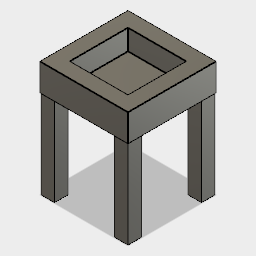
box_model_v1 (Autodesk Fusion 360 design; units mm, degrees)
Autodesk Fusion 360 part; units mm, degrees
sketch "Sketch1" plane through (0, 0, 0) normal (0, 1, 0) x (1, 0, 0)
  line L0 (14.6204, -9.8795) -> (79.6204, -9.8795)
  line L1 (79.6204, -9.8795) -> (79.6204, -74.8795)
  line L2 (79.6204, -74.8795) -> (14.6204, -74.8795)
  line L3 (14.6204, -74.8795) -> (14.6204, -9.8795)
  line L4 (68.3204, -63.5795) -> (25.9204, -63.5795)
  line L5 (25.9204, -63.5795) -> (25.9204, -21.1795)
  line L6 (25.9204, -21.1795) -> (68.3204, -21.1795)
  line L7 (68.3204, -21.1795) -> (68.3204, -63.5795)
  line L8 (15.1804, -10.4395) -> (25.1804, -10.4395)
  line L9 (25.1804, -10.4395) -> (25.1804, -20.4395)
  line L10 (25.1804, -20.4395) -> (15.1804, -20.4395)
  line L11 (15.1804, -20.4395) -> (15.1804, -10.4395)
  line L12 (79.0604, -10.4395) -> (69.0604, -10.4395)
  line L13 (69.0604, -10.4395) -> (69.0604, -20.4395)
  line L14 (69.0604, -20.4395) -> (79.0604, -20.4395)
  line L15 (79.0604, -20.4395) -> (79.0604, -10.4395)
  line L16 (15.1804, -74.3195) -> (25.1804, -74.3195)
  line L17 (25.1804, -74.3195) -> (25.1804, -64.3195)
  line L18 (25.1804, -64.3195) -> (15.1804, -64.3195)
  line L19 (15.1804, -64.3195) -> (15.1804, -74.3195)
  line L20 (79.0604, -74.3195) -> (69.0604, -74.3195)
  line L21 (69.0604, -74.3195) -> (69.0604, -64.3195)
  line L22 (69.0604, -64.3195) -> (79.0604, -64.3195)
  line L23 (79.0604, -64.3195) -> (79.0604, -74.3195)
  line L24 (17.6804, -12.9395) -> (22.6804, -12.9395)
  line L25 (22.6804, -12.9395) -> (22.6804, -17.9395)
  line L26 (22.6804, -17.9395) -> (17.6804, -17.9395)
  line L27 (17.6804, -17.9395) -> (17.6804, -12.9395)
  line L28 (76.5604, -12.9395) -> (71.5604, -12.9395)
  line L29 (71.5604, -12.9395) -> (71.5604, -17.9395)
  line L30 (71.5604, -17.9395) -> (76.5604, -17.9395)
  line L31 (76.5604, -17.9395) -> (76.5604, -12.9395)
  line L32 (17.6804, -66.8195) -> (17.6804, -71.8195)
  line L33 (17.6804, -71.8195) -> (22.6804, -71.8195)
  line L34 (22.6804, -71.8195) -> (22.6804, -66.8195)
  line L35 (22.6804, -66.8195) -> (17.6804, -66.8195)
  line L36 (76.5604, -66.8195) -> (76.5604, -71.8195)
  line L37 (76.5604, -71.8195) -> (71.5604, -71.8195)
  line L38 (71.5604, -71.8195) -> (71.5604, -66.8195)
  line L39 (71.5604, -66.8195) -> (76.5604, -66.8195)
  dimension "d1" = 65
  dimension "d2" = 65
  dimension "d6" = 11.3
  dimension "d8" = 10
  dimension "d9" = 10
  dimension "d10" = 10
  dimension "d11" = 10
  dimension "d12" = 10
  dimension "d13" = 10
  dimension "d14" = 10
  dimension "d15" = 10
  dimension "d16" = 2.5
  dimension "d17" = 2.5
  dimension "d18" = 2.5
  dimension "d19" = 2.5
  measures "d1" distance of L0.start L0.end
  measures "d2" distance of L0.start L2.end
  measures "d8" distance of L8.start L8.end
  measures "d9" distance of L8.start L10.end
  measures "d10" distance of L12.start L12.end
  measures "d11" distance of L12.start L14.end
  measures "d12" distance of L16.start L16.end
  measures "d13" distance of L16.start L18.end
  measures "d14" distance of L20.start L20.end
  measures "d15" distance of L20.start L22.end
extrude "Extrude1" add sketch "Sketch1" along normal blind 5 contours L4 L5 L6 L7 makes body 1
extrude "Extrude2" add sketch "Sketch1" along normal blind 20 contours L0 L1 L2 L3 | L8 L9 L10 L11 | L12 L13 L14 L15 | L16 L17 L18 L19 | L20 L21 L22 L23 | L24 L25 L26 L27 | L28 L29 L30 L31 | L32 L33 L34 L35 | L36 L37 L38 L39 bodies 1
extrude "Extrude3" cut sketch "Sketch1" along normal blind 3 contours L24 L25 L26 L27 | L28 L29 L30 L31 | L32 L33 L34 L35 | L36 L37 L38 L39 bodies 1
extrude "Extrude4" cut sketch "Sketch1" along normal blind 1 contours L8 L9 L10 L11 | L12 L13 L14 L15 | L16 L17 L18 L19 | L20 L21 L22 L23 bodies 1
fillet "Fillet1" radius 0.3 20 edges at (47.1204, 20, 74.8795) (79.6204, 10, 74.8795) (79.6204, 20, 42.3795) (79.6204, 10, 9.8795) (47.1204, 20, 9.8795) (14.6204, 20, 42.3795) (47.1204, 20, 63.5795) (25.9204, 20, 42.3795) (47.1204, 20, 21.1795) (68.3204, 20, 42.3795) (47.1204, 5, 63.5795) (25.9204, 5, 42.3795) (47.1204, 5, 21.1795) (68.3204, 12.5, 21.1795) (68.3204, 5, 42.3795) (68.3204, 12.5, 63.5795) (25.9204, 12.5, 63.5795) (25.9204, 12.5, 21.1795) (14.6204, 10, 74.8795) (14.6204, 10, 9.8795) on bodies 1
copy_body "Body->Comp1" bodies 1 removing the originals makes body 2 in component "Motor Housing"
sketch "Sketch2" plane through (0, 0, 0) normal (0, 1, 0) x (1, 0, 0) in component "Motor Housing"
  line L0 (100.3048, -10.6918) -> (166.3048, -10.6918)
  line L1 (166.3048, -10.6918) -> (166.3048, -20.6918)
  line L2 (166.3048, -20.6918) -> (100.3048, -20.6918)
  line L3 (100.3048, -20.6918) -> (100.3048, -10.6918)
  line L4 (100.3048, -30.5722) -> (166.3048, -30.5722)
  line L5 (166.3048, -30.5722) -> (166.3048, -40.5722)
  line L6 (166.3048, -40.5722) -> (100.3048, -40.5722)
  line L7 (100.3048, -40.5722) -> (100.3048, -30.5722)
  line L8 (100.3048, -49.9678) -> (166.3048, -49.9678)
  line L9 (166.3048, -49.9678) -> (166.3048, -59.9678)
  line L10 (166.3048, -59.9678) -> (100.3048, -59.9678)
  line L11 (100.3048, -59.9678) -> (100.3048, -49.9678)
  line L12 (100.3048, -70.0907) -> (166.3048, -70.0907)
  line L13 (166.3048, -70.0907) -> (166.3048, -80.0907)
  line L14 (166.3048, -80.0907) -> (100.3048, -80.0907)
  line L15 (100.3048, -80.0907) -> (100.3048, -70.0907)
  dimension "d32" = 66
  dimension "d33" = 10
  dimension "d34" = 10
  dimension "d35" = 10
  dimension "d36" = 10
  measures "d32" distance of L0.start L0.end
  measures "d33" distance of L0.start L2.end
  measures "d34" distance of L4.start L6.end
  measures "d35" distance of L8.start L10.end
  measures "d36" distance of L12.start L14.end
extrude "Extrude1'" add sketch "Sketch2" along normal blind 10 separate body makes body 3 at (122.3048, 3.3333, 49.9678) makes body 4 at (122.3048, 3.3333, 30.5722) makes body 5 at (122.3048, 3.3333, 70.0907) makes body 6 at (122.3048, 3.3333, 10.6918) in component "Motor Housing"
sketch "Sketch3" plane through (166.3048, 0, 0) normal (1, 0, 0) x (0, 0, -1) in component "Motor Housing"
  line L0 (-80.0907, 0) -> (-70.0907, 0)
  line L1 (-70.0907, 0) -> (-70.0907, 10)
  line L2 (-70.0907, 10) -> (-80.0907, 10)
  line L3 (-80.0907, 10) -> (-80.0907, 0)
  line L4 (-77.5907, 2.5) -> (-72.5907, 2.5)
  line L5 (-72.5907, 2.5) -> (-72.5907, 7.5)
  line L6 (-72.5907, 7.5) -> (-77.5907, 7.5)
  line L7 (-77.5907, 7.5) -> (-77.5907, 2.5)
  dimension "d39" = 2.5
sketch "Sketch4" plane through (166.3048, 0, 0) normal (1, 0, 0) x (0, 0, -1) in component "Motor Housing"
  line L0 (-59.9678, 0) -> (-49.9678, 0)
  line L1 (-49.9678, 0) -> (-49.9678, 10)
  line L2 (-49.9678, 10) -> (-59.9678, 10)
  line L3 (-59.9678, 10) -> (-59.9678, 0)
  line L4 (-57.4678, 2.5) -> (-52.4678, 2.5)
  line L5 (-52.4678, 2.5) -> (-52.4678, 7.5)
  line L6 (-52.4678, 7.5) -> (-57.4678, 7.5)
  line L7 (-57.4678, 7.5) -> (-57.4678, 2.5)
  dimension "d40" = 2.5
sketch "Sketch5" plane through (166.3048, 0, 0) normal (1, 0, 0) x (0, 0, -1) in component "Motor Housing"
  line L0 (-40.5722, 0) -> (-30.5722, 0)
  line L1 (-30.5722, 0) -> (-30.5722, 10)
  line L2 (-30.5722, 10) -> (-40.5722, 10)
  line L3 (-40.5722, 10) -> (-40.5722, 0)
  line L4 (-38.0722, 2.5) -> (-33.0722, 2.5)
  line L5 (-33.0722, 2.5) -> (-33.0722, 7.5)
  line L6 (-33.0722, 7.5) -> (-38.0722, 7.5)
  line L7 (-38.0722, 7.5) -> (-38.0722, 2.5)
  dimension "d41" = 2.5
sketch "Sketch6" plane through (166.3048, 0, 0) normal (1, 0, 0) x (0, 0, -1) in component "Motor Housing"
  line L0 (-20.6918, 0) -> (-10.6918, 0)
  line L1 (-10.6918, 0) -> (-10.6918, 10)
  line L2 (-10.6918, 10) -> (-20.6918, 10)
  line L3 (-20.6918, 10) -> (-20.6918, 0)
  line L4 (-18.1918, 2.5) -> (-13.1918, 2.5)
  line L5 (-13.1918, 2.5) -> (-13.1918, 7.5)
  line L6 (-13.1918, 7.5) -> (-18.1918, 7.5)
  line L7 (-18.1918, 7.5) -> (-18.1918, 2.5)
  dimension "d42" = 2.5
extrude "Extrude2'" add sketch "Sketch5" sketch "Sketch4" sketch "Sketch3" sketch "Sketch6" along normal blind 2 contours L4 L5 L6 L7 of sketch 2 contours L4 L5 L6 L7 of sketch 3 contours L4 L5 L6 L7 of sketch 4 contours L4 L5 L6 L7 bodies 3 4 5 6 in component "Motor Housing"
copy_body "Body->Comp1'" bodies 3 removing the originals makes body 7 in component "Leg"
copy_body "CopyPasteBodies4" bodies 5 makes body 8 in component "Motor Housing"
move_body "Move4" bodies 8 to x (1, 0, 0) y (0, 1, 0) z (0, 0, 1) at (0, 0, -20) in component "Motor Housing"
copy_body "Body->Comp3" bodies 5 removing the originals makes body 9 in component "Leg 1"
copy_body "Body->Comp4" bodies 8 removing the originals makes body 10 in component "Leg 2"
copy_body "Body->Comp5" bodies 4 removing the originals makes body 11 in component "Leg 3"
copy_body "Body->Comp6" bodies 6 removing the originals makes body 12 in component "Leg 4"
copy_body "Body->Comp7" bodies 2 removing the originals makes body 13 in component "Main Body"
component "Motor Housing" placed x (1, 0, 0) y (0, 1, 0) z (0, 0, 1) at (0, 0, 0)
component "Leg 1" placed x (0, 1, 0) y (-1, 0, 0) z (0, 0, 1) at (79.0604, -165.3048, -59.6512) in component "Motor Housing"
component "Leg 2" placed x (0, 1, 0) y (-1, 0, 0) z (0, 0, 1) at (79.0604, -165.3048, 14.2288) in component "Motor Housing"
component "Leg 3" placed x (0, 1, 0) y (-1, 0, 0) z (0, 0, 1) at (25.1804, -165.3048, -20.1327) in component "Motor Housing"
component "Leg 4" placed x (0, 1, 0) y (-1, 0, 0) z (0, 0, 1) at (25.1804, -165.3048, 53.6277) in component "Motor Housing"
component "Main Body" placed x (1, 0, 0) y (0, 1, 0) z (0, 0, 1) at (0, 0, 0) in component "Motor Housing"
